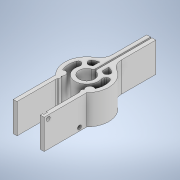
# Autodesk Inventor part: Part7
Saved by Autodesk Inventor 2021 (Build 250183000, 183)
## iProperties
Created: 2021-10-11
Part Number: Part7
Material: Generic
Document SubType Name: Modeling
Designer: Route
Density: 1 g/cm^3
Appearance: Default
Author: Route
Autodesk Inventor part; units mm, degrees
ref_plane "YZ Plane" through (0, 0, 0) normal (1, 0, 0) x (0, 1, 0)
ref_plane "XZ Plane" through (0, 0, 0) normal (0, 1, 0) x (-1, 0, 0)
ref_plane "XY Plane" through (0, 0, 0) normal (0, 0, 1) x (1, 0, 0)
sketch "Sketch1" plane through (0, 0, 0) normal (0, 1, 0) x (-1, 0, 0)
  line L0 (3, 0) -> (3, -26.9193)
  line L1 (0, -30) -> (0, 0)
  line L2 (3, 0) -> (3, 3)
  line L3 (3, 3) -> (0, 3)
  line L4 (0, 3) -> (0, 0)
  line L5 (21, 0) -> (21, -26.9193)
  line L6 (23.8993, -30) -> (23.8993, -0.0434)
  line L7 (21, 0) -> (21, 3)
  line L8 (21, 3) -> (23.8993, 3)
  line L9 (23.8993, 3) -> (23.8993, -0.0434)
  line L10 (20.6088, -28.1075) -> (20.4284, -28.3517)
  line L11 (3.3912, -28.1075) -> (3.5716, -28.3517)
  arc A0 (13.875, -47.6995) -> (10.125, -47.6995) centre (12, -42) ccw
  line L12 (12.5, -49.5993) -> (12.5, -92)
  line L13 (12.5, -92) -> (15.5, -92)
  line L14 (11.5, -49.5993) -> (11.5, -92)
  line L15 (11.5, -92) -> (8.5, -92)
  arc A1 (0, -29.9584) -> (3.5, -56.7224) centre (12, -42) ccw
  arc A2 (20.5, -56.7224) -> (23.8993, -29.8589) centre (12, -42) ccw
  line L16 (15.5, -92) -> (15.5, -65.3827)
  line L17 (15.5, -55.5554) -> (15.5, -50.2916)
  line L18 (8.5, -92) -> (8.5, -65.3827)
  line L19 (8.5, -55.5554) -> (8.5, -50.2916)
  arc A3 (20.9024, -31.195) -> (20.7826, -31.0974) centre (12, -42) ccw
  line L20 (19.6249, -49.9324) -> (20.2507, -50.7171)
  line L21 (23.8993, -51.3801) -> (24.2551, -51.0964)
  line L22 (21.5685, -47.7276) -> (20.8413, -46.8158)
  arc A4 (15.5, -55.5554) -> (19.8016, -53.6248) centre (12, -42) ccw
  arc A5 (24.9875, -47.2274) -> (24.5925, -35.8822) centre (12, -42) ccw
  arc A6 (15.5, -50.2916) -> (16.9592, -49.5104) centre (12, -42) ccw
  line L23 (4.3751, -49.9324) -> (3.7493, -50.7171)
  line L24 (2.4315, -47.7276) -> (3.1587, -46.8158)
  arc A7 (20.5132, -44.9199) -> (3.4868, -44.9199) centre (12, -42) ccw
  arc A8 (7.0408, -49.5104) -> (8.5, -50.2916) centre (12, -42) ccw
  arc A9 (4.1984, -53.6248) -> (8.5, -55.5554) centre (12, -42) ccw
  arc A10 (3.2174, -31.0974) -> (3.0976, -31.195) centre (12, -42) ccw
  arc A11 (-0.5925, -35.8822) -> (-0.9875, -47.2274) centre (12, -42) ccw
  arc A12 (20.5, -56.7224) -> (15.5, -65.3827) centre (25.5, -65.3827) ccw
  arc A13 (8.5, -65.3827) -> (3.5, -56.7224) centre (-1.5, -65.3827) ccw
  arc A14 (7.0408, -49.5104) -> (4.3751, -49.9324) centre (5.9387, -51.1794) ccw
  arc A15 (3.1587, -46.8158) -> (3.4868, -44.9199) centre (1.595, -45.5688) ccw
  arc A16 (-0.9875, -47.2274) -> (2.4315, -47.7276) centre (0.8679, -46.4806) ccw
  arc A17 (3.7493, -50.7171) -> (4.1984, -53.6248) centre (5.3129, -51.9641) ccw
  arc A18 (19.6249, -49.9324) -> (16.9592, -49.5104) centre (18.0613, -51.1794) ccw
  arc A19 (21.5685, -47.7276) -> (24.9875, -47.2274) centre (23.1321, -46.4806) ccw
  arc A20 (19.8016, -53.6248) -> (20.2507, -50.7171) centre (18.6871, -51.9641) ccw
  arc A21 (20.5132, -44.9199) -> (20.8413, -46.8158) centre (22.405, -45.5688) ccw
  arc A22 (3.2174, -31.0974) -> (3.5716, -28.3517) centre (1.9628, -29.5399) ccw
  arc A23 (20.4284, -28.3517) -> (20.7826, -31.0974) centre (22.0372, -29.5399) ccw
  arc A24 (20.6088, -28.1075) -> (21, -26.9193) centre (19, -26.9193) ccw
  arc A25 (3, -26.9193) -> (3.3912, -28.1075) centre (5, -26.9193) ccw
  arc A26 (13.875, -47.6995) -> (12.5, -49.5993) centre (14.5, -49.5993) ccw
  arc A27 (11.5, -49.5993) -> (10.125, -47.6995) centre (9.5, -49.5993) ccw
  arc A28 (20.9024, -31.195) -> (24.5925, -35.8822) centre (23, -33.3397) ccw
  arc A29 (-0.5925, -35.8822) -> (3.0976, -31.195) centre (1, -33.3397) ccw
  point P0 (19.2111, -30)
  point P1 (4.7889, -30)
  point P2 (12.5, -47.9791)
  point P3 (11.5, -47.9791)
  point P4 (8.5, -58.6358)
  point P5 (15.5, -58.6358)
  point P6 (18.3696, -48.3583)
  point P7 (21.4999, -52.2835)
  point P8 (23.4384, -50.0724)
  point P9 (20.1111, -45.9001)
  point P10 (5.6304, -48.3583)
  point P11 (2.5001, -52.2835)
  point P12 (0.5616, -50.0724)
  point P13 (3.8889, -45.9001)
  dimension "d4" = 3
  dimension "d6" = 3
  dimension "d7" = 3
  dimension "d8" = 90
  dimension "d9" = 10
  dimension "d10" = 2
  dimension "d11" = 2
  dimension "d12" = 2
  dimension "d13" = 6
  dimension "d14" = 6
  constraints: 74 point on circle, 50 end point, 32 tangent, 30 centre point, 19 point on line, 12 equal radius, 7 perpendicular, 3 coincident, 1 collinear, 1 parallel, 1 vertical
  measures "d4" distance of L12.end L13.end
  measures "d6" distance of L14.end L15.end
  measures "d7" distance of point (21.5, -52.284) L21.end
  measures "d8" angle of L22 L21
  measures "d9" radius of A12
  measures "d10" radius of A14
  measures "d11" radius of A18
  measures "d12" radius of A26
  measures "d13" diameter of A28
  measures "d14" diameter of A29
extrude "Extrusion1" add sketch "Sketch1" along normal blind 23
sketch "Sketch3" plane through (-3, 0, -26.9193) normal (-1, 0, 0) x (0, 0, 1)
  line L0 (0, 23) -> (29.9193, 23) projected
  line L1 (29.9193, 23) -> (15.7246, 23)
  circle A0 centre (26.7681, 20.3773) radius 1.5
  circle A1 centre (26.7681, 20.3773) radius 3
  circle A2 centre (2.6381, 2.5973) radius 1.5
  circle A3 centre (2.6381, 2.5973) radius 3
  point P0 (26.9193, 0)
  point P1 (1.7246, 22.9923)
  point P2 (26.9193, 46)
  point P3 (1.7246, 23.0077)
  constraints: 4 centre point, 2 coincident, 2 end point, 2 symmetric about line, 1 point on line
extrude "Extrusion2" cut sketch "Sketch3" against normal blind 1 contours A1 L0 | L0 A1 | A0 | A2 | A3
extrude "Extrusion3" cut sketch "Sketch3" against normal blind 3 contours A0 | A2
body "Solid1"
